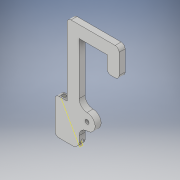
# Autodesk Inventor part: CLB_079_ScissorHookV2
Saved by Autodesk Inventor 2018 (Build 220112000, 112)
## iProperties
Created: 2020-02-08
Part Number: CLB_079_ScissorHookV2
Material: Generic
Document SubType Name: Modeling
Designer: Cooper
Density: 1 g/cm^3
Appearance: Default
Mass: 51.7458 g
Surface Area: 171.419 cm^2
Volume: 51.7458 cm^3
Author: Cooper
Autodesk Inventor part; units mm, degrees
ref_plane "YZ Plane" through (0, 0, 0) normal (1, 0, 0) x (0, 1, 0)
ref_plane "XZ Plane" through (0, 0, 0) normal (0, 1, 0) x (-1, 0, 0)
sketch "Sketch1" plane through (0, 0, 0) normal (0, 0, 1) x (1, 0, 0)
  line L0 (0, 0) -> (12.7, 0)
  line L1 (12.7, 0) -> (38.1, 25.4)
  line L2 (38.1, 25.4) -> (38.1, 38.1)
  arc A0 (50.8, 50.8) -> (38.1, 38.1) centre (50.8, 38.1) ccw
  line L3 (0, 0) -> (0, 76.2)
  line L4 (0, 76.2) -> (19.05, 76.2)
  line L5 (19.05, 190.5) -> (19.05, 76.2)
  line L6 (38.1, 171.45) -> (38.1, 88.9)
  arc A1 (50.8, 50.8) -> (50.8, 76.2) centre (50.8, 63.5) ccw
  arc A2 (38.1, 88.9) -> (50.8, 76.2) centre (50.8, 88.9) ccw
  line L7 (19.05, 190.5) -> (101.6, 190.5)
  line L8 (82.55, 171.45) -> (38.1, 171.45)
  line L9 (101.6, 190.5) -> (101.6, 146.05)
  line L10 (101.6, 146.05) -> (82.55, 146.05)
  line L11 (82.55, 146.05) -> (82.55, 171.45)
  dimension "d1" = 25.4
  dimension "d2" = 25.4
  dimension "d3" = 12.7
  dimension "d38" = 76.2
  dimension "d41" = 38.1
  dimension "d84" = 12.7
  dimension "d85" = 12.7
  dimension "d87" = 0
  dimension "d88" = 12.7
  dimension "d90" = 19.05
  dimension "d100" = 19.05
  dimension "d101" = 19.05
  dimension "d102" = 19.05
  dimension "d103" = 107.95
  dimension "d104" = 44.45
  dimension "d105" = 25.4
  constraints: 24 end point, 6 point on circle, 6 vertical, 4 horizontal, 4 tangent, 3 centre point, 1 perpendicular
  measures "d1" horizontal distance of L0.end L1.end
  measures "d2" horizontal distance of L0.end L1.end
  measures "d3" radius of A0
  measures "d38" distance between parallel lines of L0 L4
  measures "d41" distance from line of A0.centre L4
  measures "d84" radius of A1
  measures "d85" radius of A2
  measures "d87" horizontal distance of A0.centre A1.centre
  measures "d88" distance from line of L6 A0.centre
  measures "d90" distance of L3.end L4.end
  measures "d100" distance between parallel lines of L6 L5
  measures "d101" distance between parallel lines of L7 L8
  measures "d102" distance between parallel lines of L9 L11
  measures "d103" distance from line of L8 A1.centre
  measures "d104" distance of L8.start L6.start
  measures "d105" distance of L10.end L8.start
extrude "Extrusion1" add sketch "Sketch1" along normal blind 9.525
sketch "Sketch3" plane through (0, 0, 9.525) normal (0, 0, 1) x (1, 0, 0)
  line L0 (0, 76.2) -> (0, 0) projected
  line L1 (0, 0) -> (12.7, 0) projected
  arc A0 (50.8, 50.8) -> (38.1, 38.1) centre (50.8, 38.1) ccw projected
  line L2 (19.05, 76.2) -> (0, 76.2) projected
  point P0 (50.8, 63.5)
  point P1 (49.53, 54.61)
  point P2 (12.7, 82.55)
  dimension "d39" = 0
  dimension "d40" = 12.7
  constraints: 2 other
  measures "d39" horizontal distance of point (50.8, 38.1) point (50.8, 63.5)
hole "Hole2" at (50.8, 63.5, 9.525) direction (0, 0, -1) diameter 6.35 end through all
sketch "Sketch7" plane through (0, 76.2, 0) normal (0, 1, 0) x (1, 0, 0)
  line L0 (0, 0) -> (0, -9.525) projected
  point P0 (9.525, -4.7625)
  dimension "d77" = 9.525
  measures "d77" distance from line of L0 point (9.525, -4.762)
ref_plane "Work Plane6" through (38.1, 25.4, 0) normal (-0.4902612, 0.8715755, 0) x (0, 0, 1)
ref_plane "Work Plane5" through (38.1, 25.4, 4.7625) normal (0.8715755, 0.4902612, 0) x (-0.4902612, 0.8715755, 0)
sketch "Sketch8" plane through (38.1, 25.4, 0) normal (-0.4902612, 0.8715755, 0) x (0, 0, 1)
  line L0 (0, 0) -> (9.525, 0) projected
  circle A0 centre (4.7625, 0) radius 2.7813
  point P0 (0, -45.6597)
  dimension "d79" = 5.5626
  constraints: 1 centre point, 1 midpoint
  measures "d79" diameter of A0
extrude "Extrusion3" cut sketch "Sketch8" along normal through all both and the other way through all
sketch "Sketch10" plane through (0, 0, 9.525) normal (0, 0, 1) x (1, 0, 0)
  circle A0 centre (50.8, 63.5) radius 3.175 projected
  line L0 (0, 0) -> (12.7, 0) projected
  line L1 (12.7, 0) -> (38.1, 25.4) projected
  line L2 (38.1, 25.4) -> (38.1, 38.1) projected
  arc A1 (50.8, 50.8) -> (38.1, 38.1) centre (50.8, 38.1) ccw projected
  arc A2 (50.8, 50.8) -> (50.8, 76.2) centre (50.8, 63.5) ccw projected
  arc A3 (38.1, 88.9) -> (50.8, 76.2) centre (50.8, 88.9) ccw projected
  line L3 (38.1, 88.9) -> (38.1, 171.45) projected
  line L4 (19.05, 190.5) -> (19.05, 76.2) projected
  line L5 (19.05, 76.2) -> (0, 76.2) projected
  line L6 (0, 76.2) -> (0, 0) projected
  line L7 (12.7, 0) -> (38.1, 25.4) projected
  line L8 (31.75, 19.05) -> (0, 19.05)
  line L9 (38.1, 171.45) -> (82.55, 171.45) projected
  line L10 (82.55, 171.45) -> (82.55, 146.05) projected
  line L11 (82.55, 146.05) -> (101.6, 146.05) projected
  line L12 (101.6, 146.05) -> (101.6, 190.5) projected
  line L13 (101.6, 190.5) -> (19.05, 190.5) projected
  dimension "d95" = 6.35
  constraints: 2 end point, 2 point on line, 1 perpendicular
  measures "d95" distance from line of L8 L1.end
extrude "Extrusion5" cut sketch "Sketch10" against normal through all contours L6 L8 L1 L0
fillet "Fillet6" radius 6.35 9 edges at (0, 76.2, 4.7625) (0, 19.05, 4.7625) (31.75, 19.05, 4.7625) (38.1, 25.4, 8.5344) (38.1, 25.4, 0.9906) (19.05, 190.5, 4.7625) (101.6, 190.5, 4.7625) (82.55, 146.05, 4.7625) (101.6, 146.05, 4.7625)
body "Solid1"
